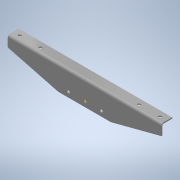
# Autodesk Inventor part: ADSK-MH-10026
Saved by Autodesk Inventor 2021.1 (Build 251245010, 245A)
## iProperties
Created: 2008-03-10
Part Number: ADSK-MH-10026
Document SubType Name: Sheet Metal
Designer: R.O'mahony
Density: 7.86 g/cm^3
Mass: 4249.93 g
Surface Area: 2270.7 cm^2
Volume: 540.703 cm^3
Material: Steel, Mild
Sheet Metal Rule: Default
Appearance: Steel
Description: Pnematic Support Bracket
Engineer: Demir Ali
Checked By: Demir Ali
Company: Autodesk Ltd
Author: R.O'mahony
Keywords: Roller Conveyor
Revision Number: A
Autodesk Inventor part; units mm, degrees
ref_plane "YZ Plane" through (0, 0, 0) normal (1, 0, 0) x (0, 1, 0)
ref_plane "XZ Plane" through (0, 0, 0) normal (0, 1, 0) x (-1, 0, 0)
ref_plane "XY Plane" through (0, 0, 0) normal (0, 0, 1) x (1, 0, 0)
sketch "Sketch1" plane through (0, 0, 0) normal (0, 0, 1) x (1, 0, 0)
  line L0 (350, -45) -> (350, -90)
  line L1 (350, -90) -> (120, -150)
  line L2 (-120, -150) -> (-350, -90)
  line L3 (-350, -90) -> (-350, -45)
  line L4 (-350, -45) -> (350, -45)
  line L5 (-350, 0) -> (350, 0)
  line L6 (350, -45) -> (350, 0)
  line L7 (-350, -45) -> (-350, 0)
  line L8 (120, -150) -> (-120, -150)
  arc A0 (2.25, -132.75) -> (2.25, -122.25) centre (2.25, -127.5) ccw
  line L9 (2.25, -122.25) -> (-2.25, -122.25)
  arc A1 (-2.25, -122.25) -> (-2.25, -132.75) centre (-2.25, -127.5) ccw
  line L10 (-2.25, -132.75) -> (2.25, -132.75)
  arc A2 (-222.75, -30.25) -> (-222.75, -19.75) centre (-222.75, -25) ccw
  line L11 (-222.75, -30.25) -> (-227.25, -30.25)
  arc A3 (-227.25, -19.75) -> (-227.25, -30.25) centre (-227.25, -25) ccw
  line L12 (-227.25, -19.75) -> (-222.75, -19.75)
  line L13 (-320, -25) -> (-225, -25) construction
  line L14 (-225, -19.75) -> (-225, -30.25) construction
  line L15 (0, -122.25) -> (0, 0) construction
  line L16 (-322.25, -25) -> (-317.75, -25) construction
  line L17 (-322.25, -30.25) -> (-317.75, -30.25)
  line L18 (-317.75, -19.75) -> (-322.25, -19.75)
  arc A4 (-322.25, -19.75) -> (-322.25, -30.25) centre (-322.25, -25) ccw
  arc A5 (-317.75, -30.25) -> (-317.75, -19.75) centre (-317.75, -25) ccw
  dimension "d7" = 4.5
  dimension "d8" = 5.25
  dimension "d9" = 22.5
  dimension "d10" = 150
  dimension "d11" = 45
  dimension "d12" = 700
  dimension "d13" = 240
  dimension "d14" = 95
  dimension "d16" = 25
  dimension "d17" = 4.5
  dimension "d18" = 30
  dimension "d19" = 2.25
  dimension "d20" = 10.5
  constraints: 40 end point, 12 point on circle, 12 tangent, 6 centre point, 6 midpoint, 6 parallel, 4 equal length, 2 collinear, 1 coincident, 1 equal radius, 1 horizontal, 1 perpendicular, 1 point on line, 1 vertical
  measures "d7" distance of A0.centre A1.centre
  measures "d8" radius of A0
  measures "d9" distance from line of L8 A0.centre
  measures "d10" distance between parallel lines of L8 L5
  measures "d11" distance between parallel lines of L4 L5
  measures "d12" distance of L5.start L5.end
  measures "d13" distance of L1.end L2.start
  measures "d14" distance of L13.start L13.end
  measures "d16" distance between parallel lines of L5 L13
  measures "d17" distance of L11.start L11.end
  measures "d18" distance from line of L7 L13.start
  measures "d19" distance of L13.start L16.end
  measures "d20" diameter of A5
extrude "Plate1" add sketch "Sketch1" along normal blind 5 contours L0 L1 L8 L2 L3 L4 | L4 L7 L5 L6 | L10 A1 L9 A0 | L11 A3 L12 A2 | A4 L18 A5 L17
extrude "Cut1" cut sketch "Sketch1" along normal blind 5 contours L11 A3 L12 A2 | A4 L18 A5 L17
extrude "Cut2" cut sketch "Sketch1" along normal blind 5 contours L10 A1 L9 A0
mirror "Mirror1" about plane through (0, 0, 0) normal (1, 0, 0) of "Cut1"
pattern_linear "Rectangular Pattern1" count 2 spacing 75 along (1, 0, 0) count 2 spacing 75 along (-1, 0, 0) of "Cut2"
fold "Fold1" angle 90 bend radius 5 thickness 5 k factor 0.44 line from (-350, -45, 0) to (350, -45, 0) line at bend centre moving side (0, -1, 0) folds toward (0, 0, -1)
equation "\"d21\" = Thickness"
equation "\"d23\" = Thickness"
equation "\"d1\" = BendReliefWidth"
equation "\"d2\" = BendReliefDepth"
equation "\"d3\" = MinimumRemnant"
equation "\"d4\" = BendRadius"
equation "\"d6\" = BendRadius"
equation "\"d31\" = Thickness"
equation "\"BendRadius\" = Thickness"
equation "\"BendReliefWidth\" = Thickness"
equation "\"BendReliefDepth\" = 0.5 * Thickness"
equation "\"TransitionRadius\" = BendRadius"
equation "\"JacobiRadiusSize\" = Thickness"
equation "\"d0\" = BendRadius"
equation "\"GapSize\" = Thickness"
equation "\"Thickness\" = 5"
equation "\"MinimumRemnant\" = 10"
body "Solid1"
